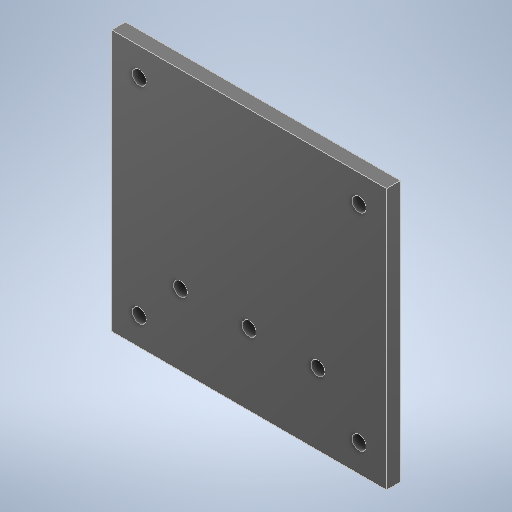
# Autodesk Inventor part: Magazine_Mount_Plate
Saved by Autodesk Inventor 2025.1 (Build 291241020, 241B)
## iProperties
Created: 2024-11-13
Part Number: Magazine_Mount_Plate
Material: PC/ABS Plastic
Document SubType Name: Modeling
Designer: leon-
Density: 1.1 g/cm^3
Appearance: Smooth - Black
Author: leon-
## iProperties of the stored document Magazine_Mount_Plate_3DPrint.ipt
Created: 2024-11-17
Part Number: Magazine_Mount_Plate_3DPrint
Material: Generic
Document SubType Name: Modeling
Designer: leon-
Density: 1 g/cm^3
Appearance: Default
Author: leon-
Autodesk Inventor part; units mm, degrees
ref_plane "YZ Plane" through (0, 0, 0) normal (1, 0, 0) x (0, 1, 0)
ref_plane "XZ Plane" through (0, 0, 0) normal (0, 1, 0) x (-1, 0, 0)
ref_plane "XY Plane" through (0, 0, 0) normal (0, 0, 1) x (1, 0, 0)
sketch "Sketch1" plane through (0, 0, 0) normal (0, 0, 1) x (1, 0, 0)
  line L0 (0, 0) -> (100, 0)
  line L1 (100, 0) -> (100, 95)
  line L2 (100, 95) -> (0, 95)
  line L3 (0, 95) -> (0, 0)
  point P0 (10, 10)
  point P1 (90, 10)
  point P2 (90, 85)
  point P3 (10, 85)
  dimension "d0" = 100
  dimension "d1" = 95
  dimension "d4" = 75
  dimension "d5" = 10
  dimension "d6" = 80
  dimension "d7" = 10
  constraints: 8 end point, 2 horizontal alignment, 2 parallel, 2 vertical alignment, 1 horizontal, 1 perpendicular
  measures "d0" distance of L1.end L2.end
  measures "d1" distance of L0.end L1.end
  measures "d4" distance of point (10, 85) point (10, 10)
  measures "d5" distance from line of L0 point (10, 10)
  measures "d6" distance of point (90, 10) point (10, 10)
  measures "d7" distance from line of L3 point (10, 10)
extrude "Extrusion1" add sketch "Sketch1" along normal blind 5
hole "Hole1" at (10, 10, 0) at (90, 10, 0) at (90, 85, 0) at (10, 85, 0) direction (0, 0, 1) diameter 5 end through all
sketch "Sketch2" plane through (0, 0, 0) normal (0, 0, -1) x (-1, 0, 0)
  line L0 (0, 95) -> (0, 0) projected
  line L1 (-100, 95) -> (0, 95) projected
  point P0 (-25, 25.901)
  point P1 (-50, 25.901)
  point P2 (-75, 25.901)
  dimension "d15" = 50
  dimension "d17" = 25
  dimension "d18" = 25
  dimension "d19" = 69.099
  constraints: 2 horizontal alignment
  measures "d15" distance from line of L0 point (-50, 25.901)
  measures "d17" distance of point (-25, 25.901) point (-50, 25.901)
  measures "d18" distance of point (-50, 25.901) point (-75, 25.901)
  measures "d19" distance from line of L1 point (-50, 25.901)
hole "Hole2" at (25, 25.901, 0) at (50, 25.901, 0) at (75, 25.901, 0) direction (0, 0, 1) diameter 5 end through all
body "Solid1"
